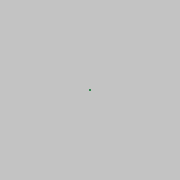
# Autodesk Inventor part: LED_colorer
Saved by Autodesk Inventor 2020 (Build 240168000, 168)
## iProperties
Created: 2019-06-06
Part Number: LED_colorer
Material: Generic
Document SubType Name: Modeling
Designer: Varga Daniel
Density: 1 g/cm^3
Appearance: Default
Author: Varga Daniel
Autodesk Inventor part; units mm, degrees
ref_plane "YZ Plane" through (0, 0, 0) normal (1, 0, 0) x (0, 1, 0)
ref_plane "XZ Plane" through (0, 0, 0) normal (0, 1, 0) x (-1, 0, 0)
ref_plane "XY Plane" through (0, 0, 0) normal (0, 0, 1) x (1, 0, 0)
sketch "Sketch1" plane through (0, 0, 0) normal (0, 0, 1) x (1, 0, 0)
  arc A0 (32.2913, 1) -> (27.7087, 1) centre (30, 0) ccw
  line L0 (32.2913, 1) -> (37.5, 1)
  line L1 (37.5, 1) -> (37.5, -1)
  line L2 (37.5, -1) -> (32.2913, -1)
  arc A1 (27.7087, -1) -> (32.2913, -1) centre (30, 0) ccw
  line L3 (27.7087, -1) -> (22.2913, -1)
  arc A2 (17.7087, -1) -> (22.2913, -1) centre (20, 0) ccw
  line L4 (17.7087, -1) -> (12.2913, -1)
  arc A3 (7.7087, -1) -> (12.2913, -1) centre (10, 0) ccw
  line L5 (7.7087, -1) -> (2.2913, -1)
  arc A4 (-2.2913, -1) -> (2.2913, -1) centre (0, 0) ccw
  line L6 (-2.2913, -1) -> (-7.5, -1)
  line L7 (-7.5, -1) -> (-7.5, 1)
  line L8 (-7.5, 1) -> (-2.2913, 1)
  arc A5 (2.2913, 1) -> (-2.2913, 1) centre (0, 0) ccw
  line L9 (2.2913, 1) -> (7.7087, 1)
  arc A6 (12.2913, 1) -> (7.7087, 1) centre (10, 0) ccw
  line L10 (12.2913, 1) -> (17.7087, 1)
  arc A7 (22.2913, 1) -> (17.7087, 1) centre (20, 0) ccw
  line L11 (22.2913, 1) -> (27.7087, 1)
  circle A8 centre (30, 0) radius 2
  circle A9 centre (10, 0) radius 2
  circle A10 centre (0, 0) radius 2
  circle A11 centre (20, 0) radius 2
  circle A12 centre (0, 0) radius 2.5
  circle A13 centre (10, 0) radius 2.5
  circle A14 centre (20, 0) radius 2.5
  circle A15 centre (30, 0) radius 2.5
  point P0 (32.2913, 1)
  point P1 (27.7087, -1)
  point P2 (27.7087, 1)
  point P3 (22.2913, 1)
  point P4 (17.7087, -1)
  point P5 (12.2913, 1)
  point P6 (7.7087, 1)
  point P7 (7.7087, 1)
  point P8 (12.2913, 1)
  point P9 (17.7087, -1)
  point P10 (22.2913, 1)
  point P11 (27.7087, 1)
  point P12 (27.7087, -1)
  point P13 (32.2913, 1)
  constraints: 24 end point, 16 centre point, 16 point on circle, 4 coincident, 4 concentric
extrude "Extrusion2" add sketch "Sketch1" along normal blind 0.1 contours A12 A4 A5 | A10
extrude "Extrusion3" add sketch "Sketch1" along normal blind 0.1 contours A13 A3 A6 | A9
extrude "Extrusion4" add sketch "Sketch1" along normal blind 0.1 contours A14 A2 A7 | A11
extrude "Extrusion5" add sketch "Sketch1" along normal blind 0.1 contours A15 A1 A0 | A8
body "Solid1"
